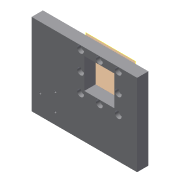
# Autodesk Inventor part: 10_Baseplate_Axiotech_mono
Saved by Autodesk Inventor 2019 (Build 230136000, 136)
## iProperties
Created: 2019-06-11
Part Number: 10_Baseplate_Axiotech_mono
Material: Generic
Document SubType Name: Modeling
Designer: diederichbenedict
Density: 1 g/cm^3
Appearance: Default
Author: diederichbenedict
Autodesk Inventor part; units mm, degrees
ref_plane "YZ Plane" through (0, 0, 0) normal (1, 0, 0) x (0, 1, 0)
ref_plane "XZ Plane" through (0, 0, 0) normal (0, 1, 0) x (-1, 0, 0)
ref_plane "XY Plane" through (0, 0, 0) normal (0, 0, 1) x (1, 0, 0)
ref_plane "Work Plane1" through (0, 0, 0) normal (0, 0, 1) x (1, 0, 0)
ref_plane "Work Plane2" through (0, 0, 0) normal (0, 0, 1) x (1, 0, 0)
sketch "Sketch3" plane through (0, 0, 0) normal (0, 0, 1) x (1, 0, 0)
  circle A0 centre (0, 25) radius 1.95 construction
  circle A1 centre (-25, 0) radius 1.95 construction
  circle A2 centre (-25, -25) radius 1.95 construction
  circle A3 centre (25, 25) radius 1.95 construction
  circle A4 centre (25, -25) radius 1.95 construction
  circle A5 centre (-25, 25) radius 1.95 construction
  circle A6 centre (25, 0) radius 1.95 construction
  circle A7 centre (0, -25) radius 1.95 construction
  line L0 (-28, 30) -> (-30, 28) construction
  line L1 (-30, 28) -> (-30, -28) construction
  line L2 (-30, -28) -> (-28, -30) construction
  line L3 (-28, -30) -> (28, -30) construction
  line L4 (28, -30) -> (30, -28) construction
  line L5 (30, -28) -> (30, 28) construction
  line L6 (30, 28) -> (28, 30) construction
  line L7 (28, 30) -> (-28, 30) construction
  line L8 (30.0525, 30.0525) -> (-79.9475, 30.0525)
  line L9 (-79.9475, 30.0525) -> (-79.9475, -29.9475)
  line L10 (-79.9475, -29.9475) -> (30.0525, -29.9475)
  line L11 (30.0525, -29.9475) -> (30.0525, 30.0525)
  line L12 (-79.9475, -29.9475) -> (-49.9475, -29.9475)
  line L13 (-49.9475, -29.9475) -> (-49.9475, -69.9475)
  line L14 (-49.9475, -69.9475) -> (-79.9475, -69.9475)
  line L15 (-79.9475, -69.9475) -> (-79.9475, -29.9475)
  point P0 (0, 0)
  dimension "d5" = 110
  dimension "d6" = 60
  dimension "d7" = 30
  dimension "d8" = 40
  constraints: 16 end point, 4 parallel, 2 horizontal, 2 perpendicular
  measures "d5" distance of L10.end L9.end
  measures "d6" distance of L9.end L8.end
  measures "d7" distance of L13.end L14.end
  measures "d8" distance of L12.end L13.end
extrude "Extrusion2" add sketch "Sketch3" along normal blind 12
sketch "Sketch4" plane through (0, 0, 12) normal (0, 0, 1) x (1, 0, 0)
  line L0 (-79.9475, 30.0525) -> (-79.9475, -69.9475) projected
  line L1 (-79.9475, -69.9475) -> (-49.9475, -69.9475) projected
  line L2 (-49.9475, -69.9475) -> (-49.9475, -29.9475) projected
  line L3 (-49.9475, -29.9475) -> (30.0525, -29.9475) projected
  line L4 (30.0525, -29.9475) -> (30.0525, 30.0525) projected
  line L5 (30.0525, 30.0525) -> (-79.9475, 30.0525) projected
  line L6 (-49.9475, -69.9475) -> (30.0525, -69.9475)
  line L7 (30.0525, -69.9475) -> (30.0525, -29.9475)
  line L8 (30.0525, -29.9475) -> (-49.9475, -29.9475)
  line L9 (-49.9475, -29.9475) -> (-49.9475, -69.9475)
  point P0 (0, 0)
  constraints: 8 end point, 2 parallel, 1 horizontal, 1 perpendicular
extrude "Extrusion3" add sketch "Sketch4" along normal blind 3
sketch "Sketch5" plane through (0, 0, 15) normal (0, 0, 1) x (1, 0, 0)
  line L0 (-79.9475, -69.9475) -> (30.0525, -69.9475) projected
  line L1 (30.0525, -69.9475) -> (30.0525, 30.0525) projected
  line L2 (30.0525, 30.0525) -> (-79.9475, 30.0525) projected
  line L3 (-79.9475, 30.0525) -> (-79.9475, -69.9475) projected
  line L4 (-79.9475, -69.9475) -> (-49.9475, -69.9475) projected
  line L5 (-79.9475, -69.9475) -> (30.0525, -69.9475)
  line L6 (30.0525, -69.9475) -> (30.0525, -78.3535)
  line L7 (30.0525, -78.3535) -> (-79.9475, -78.3535)
  line L8 (-79.9475, -78.3535) -> (-79.9475, -69.9475)
  line L9 (30.0525, -78.3535) -> (34.0525, -78.3535)
  line L10 (34.0525, -78.3535) -> (34.0525, -24.0007)
  line L11 (34.0525, -24.0007) -> (30.0525, -24.0007)
  line L12 (30.0525, -24.0007) -> (30.0525, -78.3535)
  point P0 (0, 0)
  dimension "d13" = 110
  dimension "d14" = 8.406
  dimension "d15" = 4
  dimension "d16" = 54.353
  constraints: 16 end point, 4 parallel, 2 horizontal, 2 perpendicular
  measures "d13" distance of L6.end L7.end
  measures "d15" distance of L11.end L10.end
extrude "Extrusion4" add sketch "Sketch5" against normal up to surface (15 mm away) contours L0 L6 L7 L8
sketch "Sketch6" plane through (0, 0, 15) normal (0, 0, 1) x (1, 0, 0)
  line L0 (30.0525, -78.3535) -> (30.0525, 30.0525) projected
  line L1 (30.0525, 30.0525) -> (-79.9475, 30.0525) projected
  line L2 (-79.9475, 30.0525) -> (-79.9475, -78.3535) projected
  line L3 (-79.9475, -78.3535) -> (30.0525, -78.3535) projected
  circle A0 centre (0, 25) radius 1.95 projected
  circle A1 centre (-25, 0) radius 1.95 projected
  circle A2 centre (-25, -25) radius 1.95 projected
  circle A3 centre (25, 25) radius 1.95 projected
  circle A4 centre (25, -25) radius 1.95 projected
  circle A5 centre (-25, 25) radius 1.95 projected
  circle A6 centre (25, 0) radius 1.95 projected
  circle A7 centre (0, -25) radius 1.95 projected
  line L4 (-28, 30) -> (-30, 28) projected
  line L5 (-30, 28) -> (-30, -28) projected
  line L6 (-30, -28) -> (-28, -30) projected
  line L7 (-28, -30) -> (28, -30) projected
  line L8 (28, -30) -> (30, -28) projected
  line L9 (30, -28) -> (30, 28) projected
  line L10 (30, 28) -> (28, 30) projected
  line L11 (28, 30) -> (-28, 30) projected
  point P0 (0, 0)
  constraints: 1 coincident
hole "Hole1" at (25, 25, 15) at (0, 25, 15) at (-25, 25, 15) at (-25, 0, 15) at (-25, -25, 15) at (0, -25, 15) at (25, -25, 15) at (25, 0, 15) direction (0, 0, -1) diameter 4.2 end through all counterbore diameter 9 counterbore depth 5
sketch "Sketch7" plane through (30.0525, -29.9475, 0) normal (1, 0, 0) x (0, 0, -1)
  line L0 (-10, 34.4475) -> (-10, 25.4475) projected
  line L1 (0, 0) -> (0, 60) projected
  line L2 (0, 60) -> (-15, 60) projected
  line L3 (-15, -48.406) -> (-15, 60) projected
  line L4 (-15, -48.406) -> (0, -48.406) projected
  line L5 (0, -48.406) -> (0, -40) projected
  line L6 (-12, -40) -> (0, -40) projected
  line L7 (-12, -40) -> (-12, 0) projected
  line L8 (0, 0) -> (-12, 0) projected
  point P0 (0, 29.9475)
extrude "Extrusion5" add sketch "Sketch7" along normal blind 10
sketch "Sketch8" plane through (40.0525, -29.9475, 0) normal (1, 0, 0) x (0, 0, -1)
  line L0 (0, 0) -> (0, 60) projected
  line L1 (0, 60) -> (-15, 60) projected
  line L2 (-15, 60) -> (-15, -48.406) projected
  line L3 (-15, -48.406) -> (0, -48.406) projected
  line L4 (0, -48.406) -> (0, -40) projected
  line L5 (0, -40) -> (-12, -40) projected
  line L6 (-12, -40) -> (-12, 0) projected
  line L7 (-12, 0) -> (0, 0) projected
  line L8 (0, 0) -> (-12, 0)
  line L9 (-12, 0) -> (-12, -40)
  line L10 (-12, -40) -> (0, -40)
  line L11 (0, -40) -> (0, 0)
  point P0 (0, 29.9475)
  constraints: 8 end point, 2 parallel, 1 horizontal, 1 perpendicular
extrude "Extrusion6" add sketch "Sketch8" along normal blind 10
sketch "Sketch10" plane through (0, 0, 0) normal (0, 0, -1) x (-1, 0, 0)
  line L0 (49.9475, -29.9475) -> (-40.0525, -29.9475) construction
  line L1 (49.9475, -69.9475) -> (49.9475, -29.9475) construction
  line L2 (49.9475, -69.9475) -> (-40.0525, -69.9475) construction
  line L3 (-40.0525, -69.9475) -> (-40.0525, -29.9475) construction
  circle A0 centre (-25, -25) radius 2.1 construction
  circle A1 centre (25, -25) radius 2.1 construction
  circle A2 centre (25, 25) radius 2.1 construction
  circle A3 centre (-25, 25) radius 2.1 construction
  circle A4 centre (0, 25) radius 2.1 construction
  circle A5 centre (25, 0) radius 2.1 construction
  circle A6 centre (0, -25) radius 2.1 construction
  circle A7 centre (-25, 0) radius 2.1 construction
  line L4 (-50.0525, 30.0525) -> (79.9475, 30.0525) construction
  line L5 (-50.0525, -78.3535) -> (-50.0525, 30.0525) construction
  line L6 (79.9475, -78.3535) -> (-50.0525, -78.3535) construction
  line L7 (79.9475, 30.0525) -> (79.9475, -78.3535) construction
  line L8 (39, -67) -> (34, -67) construction
  line L9 (34, -71) -> (34, -67) construction
  line L10 (34, -71) -> (39, -71) construction
  line L11 (39, -67) -> (39, -71) construction
  line L12 (28.1949, -69.9475) -> (49.9475, -69.9475)
  line L13 (49.9475, -69.9475) -> (49.9475, -73.7985)
  line L14 (49.9475, -73.7985) -> (28.1949, -73.7985)
  line L15 (28.1949, -73.7985) -> (28.1949, -69.9475)
  point P0 (0, 0)
  constraints: 8 end point, 2 parallel, 1 horizontal, 1 perpendicular, 1 point on line
extrude "Extrusion8" cut sketch "Sketch10" against normal up to surface (12 mm away)
sketch "Sketch12" plane through (-79.9475, 30.0525, 0) normal (-1, 0, 0) x (0, 0, 1)
  line L0 (10, -97.0525) -> (10, -65.0525) projected
  line L1 (0, 0) -> (0, -108.406) projected
  line L2 (15, -108.406) -> (0, -108.406) projected
  line L3 (15, 0) -> (15, -108.406) projected
  line L4 (0, 0) -> (15, 0) projected
  point P0 (0, -30.0525)
extrude "Extrusion9" add sketch "Sketch12" along normal blind 10
sketch "Sketch15" plane through (0, 0, 0) normal (0, 0, -1) x (-1, 0, 0)
  circle A0 centre (0, 0) radius 7.5 projected
  line L0 (20, -20) -> (-20, -20)
  line L1 (-20, -20) -> (-20, 20)
  line L2 (-20, 20) -> (20, 20)
  line L3 (20, 20) -> (20, -20)
  line L4 (20, -20) -> (-20, 20) construction
  line L5 (-20, -20) -> (20, 20) construction
  point P0 (0, 0)
  dimension "d52" = 40
  dimension "d53" = 40
  constraints: 12 end point, 2 midpoint, 2 parallel, 1 horizontal, 1 perpendicular
  measures "d52" distance of L1.end L2.end
  measures "d53" distance of L0.end L1.end
extrude "Extrusion10" cut sketch "Sketch15" against normal through all contours A0 | L0 L1 L2 L3
sketch "Sketch16" plane through (0, 0, 0) normal (0, 0, -1) x (-1, 0, 0)
  circle A0 centre (65.0475, -49.3535) radius 8.5 construction
  line L0 (79.9475, -68.3535) -> (79.9475, -37.8535) construction
  line L1 (79.9475, -37.8535) -> (53.5475, -37.8535) construction
  line L2 (53.5475, -37.8535) -> (53.5475, -68.3535) construction
  line L3 (53.5475, -68.3535) -> (79.9475, -68.3535) construction
  line L4 (51.5475, -35.8535) -> (81.9475, -35.8535)
  line L5 (81.9475, -35.8535) -> (81.9475, -70.3535)
  line L6 (81.9475, -70.3535) -> (51.5475, -70.3535)
  line L7 (51.5475, -70.3535) -> (51.5475, -35.8535)
  point P0 (0, 0)
  dimension "d56" = 2
  constraints: 8 end point, 3 other
  measures "d56" distance between parallel lines of L1 L4
ref_plane "Work Plane3" through (-75.6975, -60.1035, 12) normal (0, 0, 1) x (1, 0, 0)
extrude "Extrusion11" cut sketch "Sketch16" against normal up to surface (12 mm away)
sketch "Sketch17" plane through (0, 0, 15) normal (0, 0, 1) x (1, 0, 0)
  circle A0 centre (-56.5475, -49.3535) radius 0.9 projected
  circle A1 centre (-69.0475, -40.0535) radius 0.9 projected
  arc A2 (-73.0475, -47.8527) -> (-73.0475, -50.8543) centre (-73.9475, -49.3535) ccw projected
  circle A3 centre (-62.5475, -58.3535) radius 0.9 projected
  point P0 (0, 0)
hole "Hole4" at (-73.9475, -49.3535, 15) at (-69.0475, -40.0535, 15) at (-56.5475, -49.3535, 15) at (-62.5475, -58.3535, 15) direction (0, 0, -1) diameter 1 depth 10 tip angle 118 counterbore diameter 3 counterbore depth 2
body "Solid2"
